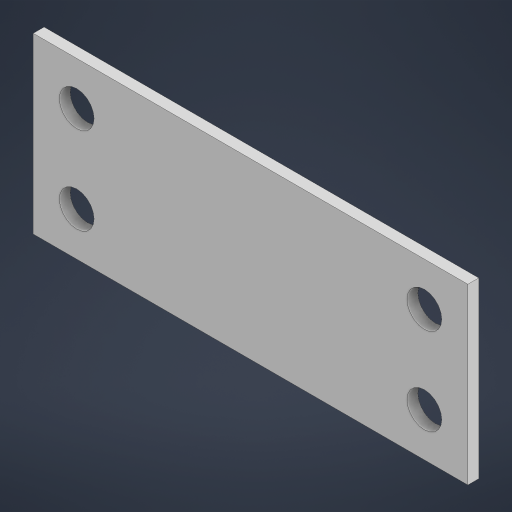
# Autodesk Inventor part: intakeRestPlate
Saved by Autodesk Inventor 2023.4 (Build 274418000, 418)
## iProperties
Created: 2024-01-28
Part Number: intakeRestPlate
Material: Generic
Document SubType Name: Modeling
Designer: Meer
Density: 1 g/cm^3
Appearance: Default
Author: Meer
Autodesk Inventor part; units mm, degrees
ref_plane "YZ Plane" through (0, 0, 0) normal (1, 0, 0) x (0, 1, 0)
ref_plane "XZ Plane" through (0, 0, 0) normal (0, 1, 0) x (-1, 0, 0)
ref_plane "XY Plane" through (0, 0, 0) normal (0, 0, 1) x (1, 0, 0)
sketch "Sketch1" plane through (0, 0, 0) normal (0, 0, 1) x (1, 0, 0)
  line L0 (0, 0) -> (63.5, 0)
  line L1 (63.5, 0) -> (63.5, 25.4)
  line L2 (63.5, 25.4) -> (0, 25.4)
  line L3 (0, 25.4) -> (0, 0)
  line L4 (3.1243, 25.4) -> (3.1243, 19.05)
  line L5 (0, 19.05) -> (6.35, 19.05)
  line L6 (6.35, 19.05) -> (57.15, 19.05)
  line L7 (57.15, 19.05) -> (57.15, 6.35)
  line L8 (57.15, 6.35) -> (6.35, 6.35)
  circle A0 centre (6.35, 19.05) radius 2.54
  circle A1 centre (57.15, 6.35) radius 2.54
  circle A2 centre (57.15, 19.05) radius 2.54
  circle A3 centre (6.35, 6.35) radius 2.54
  dimension "d0" = 63.5
  dimension "d1" = 25.4
  dimension "d2" = 6.35
  dimension "d3" = 6.35
  dimension "d4" = 50.8
  dimension "d5" = 12.7
  dimension "d6" = 5.08
  dimension "d7" = 5.08
  dimension "d8" = 5.08
  dimension "d9" = 5.08
  constraints: 18 end point, 5 perpendicular, 4 centre point, 4 coincident, 3 point on line, 2 parallel, 1 horizontal
  measures "d0" distance of L2.end L1.end
  measures "d1" distance of L0.end L1.end
  measures "d2" distance of L4.start L4.end
  measures "d3" distance of L5.start L5.end
  measures "d4" distance of L5.end L6.end
  measures "d5" distance of L6.end L7.end
  measures "d6" diameter of A0
  measures "d7" diameter of A1
  measures "d8" diameter of A2
  measures "d9" diameter of A3
extrude "Extrusion1" add sketch "Sketch1" along normal blind 1.5875
body "Solid1"
